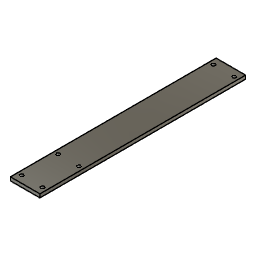
Sliding block spacer v1 (Autodesk Fusion 360 design; units mm, degrees)
Autodesk Fusion 360 part; units mm, degrees
sketch "Sketch1" plane through (0, 0, 0) normal (0, 0, 1) x (1, 0, 0)
  line L0 (17, 118.5) -> (-17, 118.5)
  line L1 (-17, 118.5) -> (-17, -118.5)
  line L2 (-17, -118.5) -> (17, -118.5)
  line L3 (17, -118.5) -> (17, 118.5)
  line L4 (17, 118.5) -> (12, 118.5)
  line L5 (12, 118.5) -> (12, 110.5) construction
  line L6 (12, 110.5) -> (17, 110.5) construction
  line L7 (17, 110.5) -> (17, 118.5)
  line L8 (-17, 118.5) -> (-12, 118.5)
  line L9 (-12, 118.5) -> (-12, 110.5) construction
  line L10 (-12, 110.5) -> (-17, 110.5) construction
  line L11 (-17, 110.5) -> (-17, 118.5)
  line L12 (-17, -118.5) -> (-12, -118.5)
  line L13 (-12, -118.5) -> (-12, -110.5) construction
  line L14 (-12, -110.5) -> (-17, -110.5) construction
  line L15 (-17, -110.5) -> (-17, -118.5)
  line L16 (17, -118.5) -> (12, -118.5)
  line L17 (12, -118.5) -> (12, -110.5) construction
  line L18 (12, -110.5) -> (17, -110.5) construction
  line L19 (17, -110.5) -> (17, -118.5)
  line L20 (12, 110.5) -> (12, 68.5) construction
  line L21 (-12, 110.5) -> (-12, 68.5) construction
  line L22 (12, -110.5) -> (12, -68.5) construction
  line L23 (-12, -110.5) -> (-12, -68.5) construction
  circle A0 centre (-12, -68.5) radius 2
  circle A1 centre (12, -68.5) radius 2
  circle A2 centre (12, -110.5) radius 2
  circle A3 centre (-12, -110.5) radius 2
  circle A4 centre (-12, 110.5) radius 2
  circle A5 centre (12, 110.5) radius 2
  dimension "d3" = 34
  dimension "d4" = 237
  dimension "d5" = 5
  dimension "d6" = 8
  dimension "d7" = 5
  dimension "d8" = 8
  dimension "d9" = 5
  dimension "d10" = 8
  dimension "d11" = 5
  dimension "d12" = 8
  dimension "d13" = 42
  dimension "d14" = 42
  dimension "d15" = 42
  dimension "d16" = 42
  dimension "d17" = 4
  dimension "d18" = 4
  dimension "d19" = 4
  dimension "d20" = 4
  dimension "d21" = 4
  dimension "d22" = 4
  constraint horizontal L0
  constraint vertical L1
  constraint horizontal L2
  constraint vertical L3
  constraint horizontal L4
  constraint vertical L5
  constraint horizontal L6
  constraint vertical L7
  constraint horizontal L8
  constraint vertical L9
  constraint horizontal L10
  constraint vertical L11
  constraint horizontal L12
  constraint vertical L13
  constraint horizontal L14
  constraint vertical L15
  constraint horizontal L16
  constraint vertical L17
  constraint horizontal L18
  constraint vertical L19
  constraint perpendicular L6 L20
  constraint perpendicular L10 L21
  constraint perpendicular L18 L22
  constraint perpendicular L14 L23
  constraint coincident L23.end A0.centre
  constraint coincident L22.end A1.centre
  constraint coincident L17.end L18.start
  constraint coincident L13.end L14.start
  constraint coincident L9.end L10.start
  constraint coincident L5.end L6.start
  measures "d3" distance of L0.start L0.end
  measures "d4" distance of L0.start L2.end
  measures "d5" distance of L0.start L4.end
  measures "d6" distance of L0.start L6.end
  measures "d7" distance of L0.end L8.end
  measures "d8" distance of L0.end L10.end
  measures "d9" distance of L1.end L12.end
  measures "d10" distance of L1.end L14.end
  measures "d11" distance of L2.end L16.end
  measures "d12" distance of L2.end L18.end
  measures "d13" distance of L5.end L20.end
  measures "d14" distance of L9.end L21.end
  measures "d15" distance of L17.end L22.end
  measures "d16" distance of L13.end L23.end
  measures "d17" diameter of A0
  measures "d18" diameter of A1
  measures "d19" diameter of A2
  measures "d20" diameter of A3
  measures "d21" diameter of A4
  measures "d22" diameter of A5
extrude "Extrude1" add sketch "Sketch1" along normal blind 4
